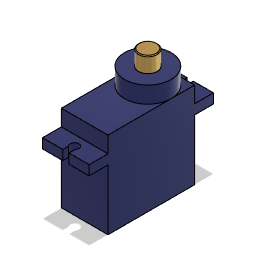
Hand v47 (Autodesk Fusion 360 archive; units mm, degrees)
design "25105 Servo"
Autodesk Fusion 360 part; units mm, degrees
sketch "Sketch1" plane through (0, 0, 0) normal (0, 1, 0) x (1, 0, 0)
  line L0 (6.05, -16.15) -> (-6.05, -16.15)
  line L1 (-6.05, -16.15) -> (-6.05, 16.15)
  line L2 (-6.05, 16.15) -> (6.05, 16.15)
  line L3 (6.05, 16.15) -> (6.05, -16.15)
  line L4 (6.05, -16.15) -> (-6.05, 16.15) construction
  line L5 (-6.05, -16.15) -> (6.05, 16.15) construction
  line L6 (6.05, -11.25) -> (-6.05, -11.25)
  line L7 (-6.05, -11.25) -> (-6.05, 11.25)
  line L8 (-6.05, 11.25) -> (6.05, 11.25)
  line L9 (6.05, 11.25) -> (6.05, -11.25)
  line L10 (6.05, -11.25) -> (-6.05, 11.25) construction
  line L11 (-6.05, -11.25) -> (6.05, 11.25) construction
  line L12 (6.05, -13.85) -> (-6.05, -13.85) construction
  line L13 (-6.05, -13.85) -> (-6.05, 13.85) construction
  line L14 (-6.05, 13.85) -> (6.05, 13.85) construction
  line L15 (6.05, 13.85) -> (6.05, -13.85) construction
  line L16 (6.05, -13.85) -> (-6.05, 13.85) construction
  line L17 (-6.05, -13.85) -> (6.05, 13.85) construction
  line L18 (0, 16.15) -> (0, -16.15) construction
  circle A0 centre (0, 13.85) radius 1.1
  circle A1 centre (0, -13.85) radius 1.1
  line L19 (0, 13.85) -> (0, 5.15)
  circle A2 centre (0, 5.15) radius 2.43
  circle A3 centre (0, 5.15) radius 6.05
  circle A4 centre (0, 5.15) radius 1
  circle A5 centre (0, -0.9) radius 2.43
  line L20 (0.8, -16.1843) -> (-0.8, -16.1843)
  line L21 (-0.8, -16.1843) -> (-0.8, -13.7157)
  line L22 (-0.8, -13.7157) -> (0.8, -13.7157)
  line L23 (0.8, -13.7157) -> (0.8, -16.1843)
  line L24 (0.8, -16.1843) -> (-0.8, -13.7157) construction
  line L25 (-0.8, -16.1843) -> (0.8, -13.7157) construction
  line L26 (0.8, 16.15) -> (-0.8, 16.15)
  line L27 (-0.8, 16.15) -> (-0.8, 13.75)
  line L28 (-0.8, 13.75) -> (0.8, 13.75)
  line L29 (0.8, 13.75) -> (0.8, 16.15)
  line L30 (0.8, 16.15) -> (-0.8, 13.75) construction
  line L31 (-0.8, 16.15) -> (0.8, 13.75) construction
  point P0 (0, -14.95)
  point P1 (0, 14.95)
  dimension "d3" = 12.1
  dimension "d4" = 32.3
  dimension "d5" = 12.1
  dimension "d6" = 22.5
  dimension "d7" = 27.7
  dimension "d8" = 2.2
  dimension "d9" = 2.2
  dimension "d10" = 8.7
  dimension "d11" = 4.86
  dimension "d12" = 2
  dimension "d23" = 4.86
  dimension "d24" = 1.6
  dimension "d25" = 1.6
  constraint horizontal L0
  constraint perpendicular L0 L1
  constraint parallel L0 L2
  constraint parallel L1 L3
  constraint coincident L4 origin
  constraint coincident L5 origin
  constraint horizontal L6
  constraint perpendicular L6 L7
  constraint parallel L6 L8
  constraint parallel L7 L9
  constraint coincident L10 origin
  constraint coincident L11 origin
  constraint horizontal L12
  constraint perpendicular L12 L13
  constraint parallel L12 L14
  constraint parallel L13 L15
  constraint coincident L16 origin
  constraint coincident L17 origin
  constraint midpoint L2 L18.start
  constraint midpoint L0 L18.end
  constraint midpoint L14 A0.centre
  constraint midpoint L12 A1.centre
  constraint coincident A0.centre L19.start
  constraint perpendicular L8 L19
  constraint coincident L19.end A2.centre
  constraint concentric A2 A3
  constraint tangent L9 A3
  constraint tangent L15 A3
  constraint concentric A3 A4
  constraint coincident A3 A5.centre
  constraint coincident L18 A5.centre
  constraint horizontal L20
  constraint perpendicular L20 L21
  constraint parallel L20 L22
  constraint parallel L21 L23
  constraint coincident L24 P0
  constraint coincident L25 P0
  constraint coincident A1 P0
  constraint coincident L18 P0
  constraint horizontal L26
  constraint perpendicular L26 L27
  constraint parallel L26 L28
  constraint parallel L27 L29
  constraint coincident L30 P1
  constraint coincident L31 P1
  constraint coincident A0 P1
  constraint coincident L18 P1
  measures "d3" distance of L1.end L2.end
  measures "d4" distance of L0.end L1.end
  measures "d5" distance of L7.end L8.end
  measures "d6" distance of L6.end L7.end
  measures "d7" distance of L12.end L13.end
  measures "d8" diameter of A0
  measures "d9" diameter of A1
  measures "d10" distance of A0.centre L19.end
  measures "d11" diameter of A2
  measures "d12" diameter of A4
  measures "d23" diameter of A5
  measures "d24" distance of L21.end L22.end
  measures "d25" distance of L27.end L28.end
extrude "Extrude1" add sketch "Sketch1" against normal blind 15.7 contours L1 L3 L6 L7 L9 A3 A5 | L3 L8 L9 L19 A3 | A3 A5 | L1 L7 L8 L19 A3 | A3 A5 | A3 A5 | A2 | A4
extrude "Extrude2" add sketch "Sketch1" along normal blind 2.5 contours L0 L1 L3 L6 A1 L21 L23 | L1 L3 L6 L7 L9 A3 A5 | L3 L8 L9 L19 A3 | A3 A5 | L2 L3 L8 A0 L19 L29 | L1 L7 L8 L19 A3 | A3 A5 | A3 A5 | L1 L2 L8 A0 L19 L27 | A2 | A4
extrude "Extrude3" add sketch "Sketch1" along normal blind 6.7 contours L1 L3 L6 L7 L9 A3 A5 | L3 L8 L9 L19 A3 | A3 A5 | L1 L7 L8 L19 A3 | A3 A5 | A3 A5 | A2 | A4
extrude "Extrude4" add sketch "Sketch1" along normal blind 11 contours A3 A5 | A3 A5 | A2 | A4 picked at (2.681, 1.8148) picked at (0.4447, -0.0905)
extrude "Extrude5" add sketch "Sketch1" along normal blind 15 contours A2 | A4
fillet "Fillet1" radius 0.2 1 edges at (-2.2656, 15, -4.2713)
equation "d15 = 18.2 mm - 15.7 mm"
equation "d17 = 22.4 mm - 15.7 mm"
equation "d19 = 26.7 mm - 15.7 mm"
equation "d21 = 30.7 mm - 15.7 mm"

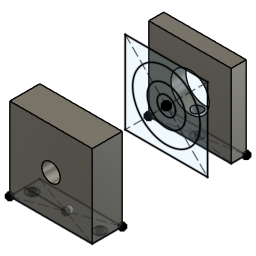
design "ThumbBrackets"
Autodesk Fusion 360 part; units mm, degrees
sketch "Sketch2" plane through (0, 0, 0) normal (0, 0, 1) x (1, 0, 0)
  circle A0 centre (0, 0) radius 2.45
  line L0 (11, 11) -> (-11, 11)
  line L1 (-11, 11) -> (-11, -11)
  line L2 (-11, -11) -> (11, -11)
  line L3 (11, -11) -> (11, 11)
  line L4 (11, 11) -> (-11, -11) construction
  line L5 (-11, 11) -> (11, -11) construction
  circle A1 centre (0, 0) radius 9
  circle A2 centre (0, 0) radius 5.1
  dimension "d17" = 4.9
  dimension "d18" = 22
  dimension "d90" = 18
  dimension "d104" = 10.2
  dimension "d121" = 22
  constraint coincident A0.centre A1.centre
  constraint horizontal L0
  constraint perpendicular L0 L1
  constraint parallel L0 L2
  constraint parallel L1 L3
  constraint coincident L4 A0.centre
  constraint coincident L5 A0.centre
  constraint concentric A0 A1
  measures "d17" diameter of A0
  measures "d18" distance of L1.end L2.end
  measures "d90" diameter of A1
  measures "d104" diameter of A2
  measures "d121" distance of L0.start L2.end
extrude "Extrude3" add sketch "Sketch2" against normal blind 4 from surface at -6.3 contours A0 | L0 L1 L2 L3 | A1 | A2 makes body 1
extrude "Extrude4" add sketch "Sketch2" along normal blind 4 from surface at 22.8 separate body contours L0 L1 L2 L3 makes body 2
extrude "Extrude5" add sketch "Sketch2" along normal blind 4 from surface at 26.8 contours L0 L1 L2 L3 | A1 | A2 bodies 2
sketch "Sketch7" plane through (0, -11, 0) normal (0, -1, 0) x (1, 0, 0)
  line L0 (-11, 22.8) -> (11, 22.8)
  line L1 (11, 22.8) -> (11, 30.8)
  line L2 (11, 30.8) -> (-11, 30.8)
  line L3 (-11, 30.8) -> (-11, 22.8)
  line L4 (11, 22.8) -> (-11, 22.8)
  line L5 (-11, 22.8) -> (-11, 30.8)
  line L6 (-11, 30.8) -> (11, 30.8)
  line L7 (11, 30.8) -> (11, 22.8)
  line L8 (11, 30.8) -> (-11, 22.8) construction
  line L9 (-11, 30.8) -> (11, 22.8) construction
  line L10 (0, 26.8) -> (-11, 26.8)
  circle A0 centre (-9, 26.8) radius 1.425
  line L11 (0, 26.8) -> (0, 26)
  circle A1 centre (9, 26.8) radius 1.425
  point P0 (0, 26.8)
  dimension "d98" = 2.85
  dimension "d99" = 9
  constraint horizontal L4
  constraint vertical L5
  constraint horizontal L6
  constraint vertical L7
  constraint coincident L2.end L3.start
  constraint coincident L0.end L1.start
  constraint midpoint L8 P0
  constraint midpoint L5 L10.end
  constraint coincident L10 A0.centre
  constraint coincident P0 L10.start
  constraint perpendicular L10 L11
  constraint symmetric A0 L11 A1
  measures "d98" diameter of A0
  measures "d99" distance of A0.centre P0
sketch "Sketch8" plane through (0, -11, 0) normal (0, -1, 0) x (1, 0, 0)
  line L0 (11, -6.3) -> (-11, -6.3)
  line L1 (-11, -6.3) -> (-11, -10.3)
  line L2 (-11, -10.3) -> (11, -10.3)
  line L3 (11, -10.3) -> (11, -6.3)
  line L4 (11, -10.3) -> (-11, -10.3)
  line L5 (-11, -10.3) -> (-11, -6.3)
  line L6 (-11, -6.3) -> (11, -6.3)
  line L7 (11, -6.3) -> (11, -10.3)
  line L8 (11, -10.3) -> (-11, -6.3) construction
  line L9 (11, -6.3) -> (-11, -10.3) construction
  circle A0 centre (0, -8.3) radius 1.425
  dimension "d72" = 2.85
  constraint horizontal L4
  constraint vertical L5
  constraint horizontal L6
  constraint vertical L7
  constraint coincident L0.end L1.start
  constraint coincident L2.end L3.start
  constraint midpoint L9 A0.centre
  measures "d72" diameter of A0
extrude "Extrude9" cut sketch "Sketch7" sketch "Sketch8" against normal blind 7 contours L10 A0 | L10 A0 | A1 of sketch 2 contours A0 bodies 1 2
extrude "Extrude11" cut sketch "Sketch2" against normal blind 10.5 contours A0 | A2 bodies 1
equation "d19 = -6 mm - 0.3 mm"
equation "d22 = 22.5 mm + 0.3 mm"
equation "d26 = 22.5 mm + 0.3 mm + 4 mm"
equation "d109 = -2 mm + 0.05 mm"

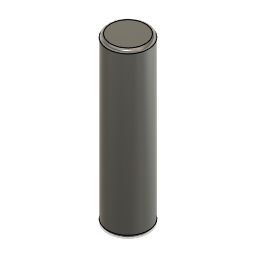
design "Finger Pin"
Autodesk Fusion 360 part; units mm, degrees
sketch "Sketch1" plane through (0, 0, 0) normal (0, 1, 0) x (1, 0, 0)
  circle A0 centre (0, 0) radius 2
  dimension "d1" = 4
  constraint coincident A0.centre origin
  measures "d1" diameter of A0
extrude "Extrude1" add sketch "Sketch1" along normal blind 16
fillet "Fillet1" radius 0.3 2 edges at (-1.8647, 16, 0.7232) (-1.8647, 0, 0.7232)

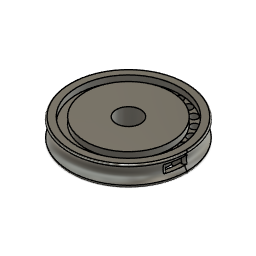
design "Servo Pulley"
Autodesk Fusion 360 part; units mm, degrees
sketch "Sketch1" plane through (0, 0, 0) normal (0, 1, 0) x (1, 0, 0)
  circle A0 centre (0, 0) radius 2.43
  dimension "d1" = 4.86
  constraint coincident A0.centre origin
  measures "d1" diameter of A0
sketch "Sketch2" plane through (0, 0, 0) normal (0, 0, 1) x (1, 0, 0)
  line L0 (0, 0) -> (12, 0)
  line L1 (12, 0) -> (12, 2) construction
  line L2 (12, 0) -> (12, -2) construction
  line L3 (12, 0) -> (11, 0)
  spline S0 degree 5 poles (12, 2) (11.924152, 1.92) (11.779081, 1.76) (11.581344, 1.52) (11.358096, 1.2) (11.150939, 0.8) (11.022111, 0.4) (10.978005, 0) (11.022111, -0.4) (11.150939, -0.8) (11.358096, -1.2) (11.581344, -1.52) (11.779081, -1.76) (11.924152, -1.92) (12, -2) knots 0 0 0 0 0 0 0.1 0.2 0.3 0.4 0.5 0.6 0.7 0.8 0.9 1 1 1 1 1 1
  line L4 (12, 2) -> (0, 2)
  line L5 (0, 2) -> (0, -2)
  line L6 (0, -2) -> (12, -2)
  line L7 (12, -2) -> (12, 2)
  line L8 (11.170521, -0.8) -> (10.170521, -0.8)
  line L9 (10.170521, -0.8) -> (10.170521, -2)
  line L10 (8.570521, -2) -> (8.570521, 0)
  line L11 (8.570521, 0) -> (8.570521, 0.8)
  line L12 (8.570521, 0.8) -> (11.170521, 0.8)
  line L13 (10.170521, -0.8) -> (10.170521, 0.8)
  line L14 (8.570521, 0.8) -> (8.570521, 2)
  line L15 (10.170521, 0.8) -> (10.170521, 2)
  dimension "d3" = 2
  dimension "d4" = 12
  dimension "d6" = 1
  dimension "d7" = 12
  dimension "d8" = 4
  dimension "d16" = 1
  dimension "d17" = 0.8
  dimension "d18" = 1.6
  dimension "d22" = 0.8
  constraint coincident L0.start origin
  constraint horizontal L0
  constraint perpendicular L0 L1
  constraint symmetric L1.start L0 L2.start
  constraint symmetric L0 L1.end L2.end
  constraint perpendicular L2 L3
  constraint horizontal L4
  constraint vertical L5
  constraint horizontal L6
  constraint vertical L7
  constraint horizontal L8
  constraint perpendicular L6 L9
  constraint perpendicular L0 L10
  constraint perpendicular L0 L11
  constraint perpendicular L11 L12
  constraint perpendicular L12 L13
  constraint perpendicular L4 L14
  constraint perpendicular L4 L15
  measures "d3" distance of L0.end L1.end
  measures "d4" distance of L0.start L0.end
  measures "d6" distance of L0.end L3.end
  measures "d7" distance of L1.end L4.end
  measures "d8" distance of L1.end L2.end
  measures "d17" distance of L0 L8
  measures "d18" distance of L9 L10
  measures "d22" distance of L0 L12
revolve "Revolve1" add sketch "Sketch2" angle 360 about axis through (0, 2, 0) along (0, -1, 0) contours L0 L4 L5 L11 L14 | L0 L5 L6 L10 | L0 L11 L12 L13 | L0 L6 L9 L10 L13 | L0 S0 L12 L13 | L0 S0 L8 L13 | L4 L12 L14 L15 | S0 L6 L8 L9 | S0 L4 L12 L15 picked at (2.85684, 0.933333) picked at (2.85684, -0.666667) picked at (9.103854, 0.533333) picked at (9.103854, -0.933333) picked at (10.453444, 0.355556) picked at (10.453444, -0.355556) picked at (9.637187, 1.2) picked at (10.572376, -1.333333) picked at (10.572376, 1.333333)
extrude "Extrude1" cut sketch "Sketch1" along normal blind 5 and the other way blind 7 contours A0 picked at (0.117604, 0.586624)
fillet "Fillet1" radius 0.25 2 edges at (-11.187928, 2, -4.339385) (-11.187928, -2, -4.339385)
revolve "Revolve2" cut sketch "Sketch2" angle 16 about axis through (0, 2, 0) along (0, -1, 0) contours L0 L11 L12 L13 | L0 L6 L9 L10 L13 | L0 S0 L12 L13 | L0 S0 L8 L13 picked at (9.103854, 0.533333) picked at (9.103854, -0.933333) picked at (10.453444, 0.355556) picked at (10.453444, -0.355556)
fillet "Fillet2" radius 0.5 2 edges at (11, 0, 0) (10.574018, -0.022212, 3.032051)
fillet "Fillet3" radius 0.15 1 edges at (10.071542, -0.8, 1.415463)
sketch "Sketch3" plane through (0, -2, 0) normal (0, -1, 0) x (1, 0, 0)
  arc A0 (10.170521, 0) -> (9.776532, 2.803375) centre (0, 0) ccw
  line L0 (10.170521, 0) -> (8.570521, 0)
  arc A1 (8.570521, 0) -> (8.238513, 2.362356) centre (0, 0) ccw
  line L1 (8.238513, 2.362356) -> (9.776532, 2.803375)
  circle A2 centre (0, 0) radius 2.43
  spline S0 degree 3 poles (11.453956, 0) (11.453956, -2.560866) (10.564266, -5.113528) (7.619304, -8.824831) (5.769819, -10.131159) (1.709075, -11.521608) (-0.483848, -11.637642) (-4.563554, -10.707343) (-6.450112, -9.68858) (-9.497493, -6.756926) (-10.617015, -4.810222) (-11.6176, -0.703675) (-11.549847, 1.436761) (-10.281544, 5.504359) (-9.011526, 7.402765) (-5.887634, 10.00107) (-4.154122, 10.836468) (-0.280254, 11.639218) (1.879119, 11.489914) (5.457781, 10.214534) (6.938543, 9.272583) (9.431509, 6.752659) (10.400789, 5.135689) (11.28087, 2.290643) (11.453956, 1.145396) (11.453956, 0) knots -6.28318531 -6.28318531 -6.28318531 -6.28318531 -5.61241784 -5.61241784 -5.04228934 -5.04228934 -4.48819863 -4.48819863 -3.94635093 -3.94635093 -3.38059974 -3.38059974 -2.83935243 -2.83935243 -2.26461057 -2.26461057 -1.77514115 -1.77514115 -1.22846068 -1.22846068 -0.78003486 -0.78003486 -0.30001341 -0.30001341 0 0 0 0
  circle A3 centre (9.19755, -1.726254) radius 0.8
  circle A4 centre (9.19755, -1.726254) radius 0.8
  circle A5 centre (8.437363, -4.047935) radius 0.8
  circle A6 centre (7.102184, -6.093755) radius 0.8
  circle A7 centre (5.283004, -7.724296) radius 0.8
  circle A8 centre (3.103795, -8.828439) radius 0.8
  circle A9 centre (0.713067, -9.330938) radius 0.8
  line L2 (0, 0) -> (11.453956, 0)
  circle A10 centre (3.103795, 8.828439) radius 0.8
  circle A11 centre (0.713067, 9.330938) radius 0.8
  circle A12 centre (5.283004, 7.724296) radius 0.8
  circle A13 centre (7.102184, 6.093755) radius 0.8
  circle A14 centre (8.437363, 4.047935) radius 0.8
  circle A15 centre (9.19755, 1.726254) radius 0.8
  circle A16 centre (0, 0) radius 8.558145
  circle A17 centre (0, 0) radius 10.158145
  dimension "d25" = 1.6
  dimension "d40" = 1.6
  dimension "d44" = -75
  constraint coincident A0.centre A1.centre
  constraint horizontal L2
  constraint symmetric A3 L2 A15
  constraint symmetric A5 L2 A14
  constraint symmetric A6 L2 A13
  constraint symmetric A7 L2 A12
  constraint symmetric A8 L2 A10
  constraint symmetric A9 L2 A11
  constraint tangent A12 A16
  constraint concentric A16 A17
  constraint tangent A12 A17
  measures "d25" diameter of A3
  measures "d40" diameter of A4
extrude "Extrude2" cut sketch "Sketch3" against normal blind 4.5 contours A3 A4 | A14 | A5 | A13 | A6 | A12 | A7 | A10 | A8 | A11 | A9 picked at (9.384011, -1.906251) picked at (8.852966, 4.197622) picked at (8.303969, -3.817227) picked at (6.742554, 6.316638) picked at (7.241812, -5.849214) picked at (5.199978, 7.863305) picked at (5.766903, -7.919166) picked at (3.321685, 9.03035) picked at (3.346725, -8.74498) picked at (0.846062, 9.099971) picked at (0.410309, -9.04431)
extrude "Extrude3" cut sketch "Sketch3" along normal blind 1.2 from surface at -4 contours L0 A3 A4 L2 A16 A17 | L0 A1 L2 A15 A17 | A1 L1 A15 A17 | A1 L1 A14 A15 A16 A17 | A1 L2 A15 A16 | A1 A15 | A3 A4 A5 A16 A17 | A3 A4 | A14 | A13 A14 A16 A17 | A1 A15 | A5 A6 A16 A17 | A5 | A13 | A12 A13 A16 A17 | A6 A7 A16 A17 | A6 | A12 | A10 A12 A16 A17 | A7 A8 A16 A17 | A7 | A10 | A10 A11 A16 A17 | A8 A9 A16 A17 | A8 | A11 | A9 A11 A16 A17 | A9 picked at (9.33344, -0.309898) picked at (9.336327, 0.310182) picked at (9.729456, 2.574804) picked at (8.910766, 2.821788) picked at (8.516723, 0.851095) picked at (9.450731, 1.829124) picked at (9.315667, -2.894906) picked at (9.384011, -1.906251) picked at (8.852966, 4.197622) picked at (8.258674, 5.221366) picked at (8.419311, 1.58019) picked at (8.258674, -5.221366) picked at (8.303969, -3.817227) picked at (6.742554, 6.316638) picked at (6.627542, 7.186336) picked at (6.627542, -7.186336) picked at (7.241812, -5.849214) picked at (5.199978, 7.863305) picked at (4.541855, 8.664167) picked at (4.541855, -8.664167) picked at (5.766903, -7.919166) picked at (3.321685, 9.03035) picked at (2.150758, 9.515148) picked at (2.150758, -9.515148) picked at (3.346725, -8.74498) picked at (0.846062, 9.099971) picked at (-4.69206, -8.126516) picked at (0.410309, -9.04431)

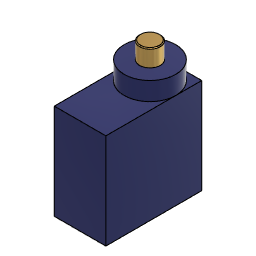
design "25105 Servo Clipped"
Autodesk Fusion 360 part; units mm, degrees
sketch "Sketch1" plane through (0, 0, 0) normal (0, 1, 0) x (1, 0, 0)
  line L0 (6.05, -16.15) -> (-6.05, -16.15)
  line L1 (-6.05, -16.15) -> (-6.05, 16.15)
  line L2 (-6.05, 16.15) -> (6.05, 16.15)
  line L3 (6.05, 16.15) -> (6.05, -16.15)
  line L4 (6.05, -16.15) -> (-6.05, 16.15) construction
  line L5 (-6.05, -16.15) -> (6.05, 16.15) construction
  line L6 (6.05, -11.25) -> (-6.05, -11.25)
  line L7 (-6.05, -11.25) -> (-6.05, 11.25)
  line L8 (-6.05, 11.25) -> (6.05, 11.25)
  line L9 (6.05, 11.25) -> (6.05, -11.25)
  line L10 (6.05, -11.25) -> (-6.05, 11.25) construction
  line L11 (-6.05, -11.25) -> (6.05, 11.25) construction
  line L12 (6.05, -13.85) -> (-6.05, -13.85) construction
  line L13 (-6.05, -13.85) -> (-6.05, 13.85) construction
  line L14 (-6.05, 13.85) -> (6.05, 13.85) construction
  line L15 (6.05, 13.85) -> (6.05, -13.85) construction
  line L16 (6.05, -13.85) -> (-6.05, 13.85) construction
  line L17 (-6.05, -13.85) -> (6.05, 13.85) construction
  line L18 (0, 16.15) -> (0, -16.15) construction
  circle A0 centre (0, 13.85) radius 1.1
  circle A1 centre (0, -13.85) radius 1.1
  line L19 (0, 13.85) -> (0, 5.15)
  circle A2 centre (0, 5.15) radius 2.43
  circle A3 centre (0, 5.15) radius 6.05
  circle A4 centre (0, 5.15) radius 1
  circle A5 centre (0, -0.9) radius 2.43
  line L20 (0.8, -16.1843) -> (-0.8, -16.1843)
  line L21 (-0.8, -16.1843) -> (-0.8, -13.7157)
  line L22 (-0.8, -13.7157) -> (0.8, -13.7157)
  line L23 (0.8, -13.7157) -> (0.8, -16.1843)
  line L24 (0.8, -16.1843) -> (-0.8, -13.7157) construction
  line L25 (-0.8, -16.1843) -> (0.8, -13.7157) construction
  line L26 (0.8, 16.15) -> (-0.8, 16.15)
  line L27 (-0.8, 16.15) -> (-0.8, 13.75)
  line L28 (-0.8, 13.75) -> (0.8, 13.75)
  line L29 (0.8, 13.75) -> (0.8, 16.15)
  line L30 (0.8, 16.15) -> (-0.8, 13.75) construction
  line L31 (-0.8, 16.15) -> (0.8, 13.75) construction
  point P0 (0, -14.95)
  point P1 (0, 14.95)
  dimension "d3" = 12.1
  dimension "d4" = 32.3
  dimension "d5" = 12.1
  dimension "d6" = 22.5
  dimension "d7" = 27.7
  dimension "d8" = 2.2
  dimension "d9" = 2.2
  dimension "d10" = 8.7
  dimension "d11" = 4.86
  dimension "d12" = 2
  dimension "d23" = 4.86
  dimension "d24" = 1.6
  dimension "d25" = 1.6
  constraint horizontal L0
  constraint perpendicular L0 L1
  constraint parallel L0 L2
  constraint parallel L1 L3
  constraint coincident L4 origin
  constraint coincident L5 origin
  constraint horizontal L6
  constraint perpendicular L6 L7
  constraint parallel L6 L8
  constraint parallel L7 L9
  constraint coincident L10 origin
  constraint coincident L11 origin
  constraint horizontal L12
  constraint perpendicular L12 L13
  constraint parallel L12 L14
  constraint parallel L13 L15
  constraint coincident L16 origin
  constraint coincident L17 origin
  constraint midpoint L2 L18.start
  constraint midpoint L0 L18.end
  constraint midpoint L14 A0.centre
  constraint midpoint L12 A1.centre
  constraint coincident A0.centre L19.start
  constraint perpendicular L8 L19
  constraint coincident L19.end A2.centre
  constraint concentric A2 A3
  constraint tangent L9 A3
  constraint tangent L15 A3
  constraint concentric A3 A4
  constraint coincident A3 A5.centre
  constraint coincident L18 A5.centre
  constraint horizontal L20
  constraint perpendicular L20 L21
  constraint parallel L20 L22
  constraint parallel L21 L23
  constraint coincident L24 P0
  constraint coincident L25 P0
  constraint coincident A1 P0
  constraint coincident L18 P0
  constraint horizontal L26
  constraint perpendicular L26 L27
  constraint parallel L26 L28
  constraint parallel L27 L29
  constraint coincident L30 P1
  constraint coincident L31 P1
  constraint coincident A0 P1
  constraint coincident L18 P1
  measures "d3" distance of L1.end L2.end
  measures "d4" distance of L0.end L1.end
  measures "d5" distance of L7.end L8.end
  measures "d6" distance of L6.end L7.end
  measures "d7" distance of L12.end L13.end
  measures "d8" diameter of A0
  measures "d9" diameter of A1
  measures "d10" distance of A0.centre L19.end
  measures "d11" diameter of A2
  measures "d12" diameter of A4
  measures "d23" diameter of A5
  measures "d24" distance of L21.end L22.end
  measures "d25" distance of L27.end L28.end
extrude "Extrude1" add sketch "Sketch1" against normal blind 15.7 contours L1 L3 L6 L7 L9 A3 A5 | L3 L8 L9 L19 A3 | A3 A5 | L1 L7 L8 L19 A3 | A3 A5 | A3 A5 | A2 | A4
extrude "Extrude2" add sketch "Sketch1" along normal blind 2.5 contours L1 L3 L6 L7 L9 A3 A5 | L3 L8 L9 L19 A3 | A3 A5 | L1 L7 L8 L19 A3 | A3 A5 | A3 A5 | A2 | A4
extrude "Extrude3" add sketch "Sketch1" along normal blind 6.7 contours L1 L3 L6 L7 L9 A3 A5 | L3 L8 L9 L19 A3 | A3 A5 | L1 L7 L8 L19 A3 | A3 A5 | A3 A5 | A2 | A4
extrude "Extrude4" add sketch "Sketch1" along normal blind 11 contours A3 A5 | A3 A5 | A2 | A4 picked at (2.681, 1.8148) picked at (0.4447, -0.0905)
extrude "Extrude5" add sketch "Sketch1" along normal blind 15 contours A2 | A4
fillet "Fillet1" radius 0.2 1 edges at (-2.2656, 15, -4.2713)
equation "d15 = 18.2 mm - 15.7 mm"
equation "d17 = 22.4 mm - 15.7 mm"
equation "d19 = 26.7 mm - 15.7 mm"
equation "d21 = 30.7 mm - 15.7 mm"
